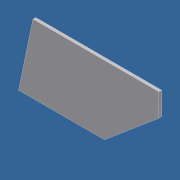
# Autodesk Inventor part: GE-12053-02
Saved by Autodesk Inventor 2012 (Build 160160000, 160)
## iProperties
Created: 2011-08-29
Part Number: GE-12053-02
Document SubType Name: Modeling
Designer: mcyr
Density: 1 g/cm^3
Description: Shelf Support
Material: Default
Title: Shelf Support
Author: mcyr
Autodesk Inventor part; units mm, degrees
ref_plane "YZ Plane" through (0, 0, 0) normal (1, 0, 0) x (0, 1, 0)
ref_plane "XZ Plane" through (0, 0, 0) normal (0, 1, 0) x (-1, 0, 0)
ref_plane "XY Plane" through (0, 0, 0) normal (0, 0, 1) x (1, 0, 0)
sketch "Sketch1" plane through (0, 0, 0) normal (0, 0, 1) x (1, 0, 0)
  line L0 (0, 0) -> (31.75, 152.4)
  line L1 (31.75, 152.4) -> (311.15, 152.4)
  line L2 (311.15, 152.4) -> (311.15, 101.6)
  line L3 (311.15, 101.6) -> (190.5, 0)
  line L4 (190.5, 0) -> (0, 0)
  dimension "d0" = 152.4
  dimension "d1" = 279.4
  dimension "d2" = 50.8
  dimension "d3" = 190.5
  dimension "d4" = 31.75
  constraints: 10 end point, 2 perpendicular, 1 horizontal
  measures "d0" distance between parallel lines of L4 L1
  measures "d1" distance of L0.end L1.end
  measures "d2" distance of L1.end L2.end
  measures "d3" distance of L3.end L0.start
  measures "d4" horizontal distance of L0.end L0.start
extrude "Extrusion1" add sketch "Sketch1" along normal blind 6.35
body "Solid1"
